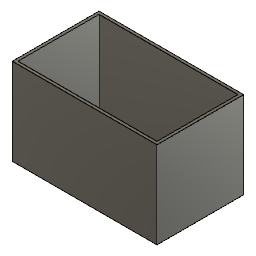
fusion_sample_file (Autodesk Fusion 360 design; units mm, degrees)
Autodesk Fusion 360 part; units mm, degrees
sketch "Sketch1" plane through (0, 0, 0) normal (0, 1, 0) x (1, 0, 0)
  line L0 (0, 0) -> (50, 0)
  line L1 (50, 0) -> (50, 30)
  line L2 (50, 30) -> (0, 30)
  line L3 (0, 30) -> (0, 0)
  line L4 (49, 29) -> (1, 29)
  line L5 (1, 29) -> (1, 1)
  line L6 (1, 1) -> (49, 1)
  line L7 (49, 1) -> (49, 29)
  dimension "d16" = 50
  dimension "d17" = 30
  constraint horizontal L0
  constraint vertical L1
  constraint horizontal L2
  constraint vertical L3
  constraint coincident L0.start L3.end
  measures "d16" distance of L0.start L0.end
  measures "d17" distance of L0.end L1.end
extrude "Extrude5" add sketch "Sketch1" along normal blind 30
extrude "Extrude6" add sketch "Sketch1" along normal blind 1 contours L4 L5 L6 L7
equation "thickness = 1 mm"
equation "depth = 30 mm"
equation "width = 50 mm"
equation "height = 30 mm"
equation "d16 = width"
equation "d17 = depth"
equation "d18 = -thickness"
equation "d19 = height"
equation "d21 = thickness"
